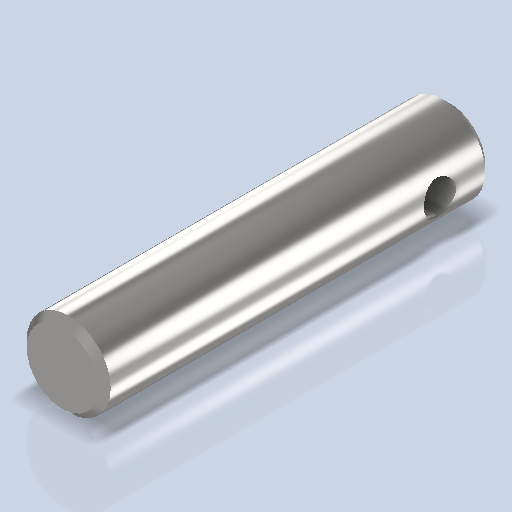
# Autodesk Inventor part: BMS_bolts
Saved by Autodesk Inventor 2024.2 (Build 282272000, 272)
## iProperties
Created: 2024-05-14
Part Number: BMS_bolts
Material: Edelstahl
Document SubType Name: Modeling
Designer: Fabri
Density: 8 g/cm^3
Appearance: Halbpoliert
Author: Fabri
Autodesk Inventor part; units mm, degrees
ref_plane "XZ Plane" through (0, 0, 0) normal (0, 1, 0) x (-1, 0, 0)
ref_plane "XY Plane" through (0, 0, 0) normal (0, 0, 1) x (1, 0, 0)
sketch "Skizze1" plane through (0, 0, 0) normal (0, 1, 0) x (-1, 0, 0)
  circle A0 centre (0, 0) radius 3.25
  dimension "d0" = 6.5
  constraints: 1 centre point, 1 coincident
  measures "d0" diameter of A0
extrude "Extrusion1" add sketch "Skizze1" along normal blind 30
chamfer "Fasen1" distance 0.5 angle 45 2 edges at (3.25, 30, 0) (3.25, 0, 0)
ref_plane "Arbeitsebene1" through (3.25, 0, 0) normal (1, 0, 0) x (0, 1, 0)
sketch "Skizze2" plane through (3.25, 0, 0) normal (1, 0, 0) x (0, 1, 0)
  line L0 (0, -2.75) -> (0, 2.75) projected
  line L1 (30, 2.75) -> (30, -2.75) projected
  point P0 (0, 0)
  point P1 (26, 0)
  point P2 (0, 0)
  dimension "d8" = 4
  constraints: 1 horizontal alignment, 1 midpoint
  measures "d8" distance from line of L1 point (26, 0)
hole "Bohrung1" at (3.25, 26, 0) direction (-1, 0, 0) diameter 2.5 end through all
